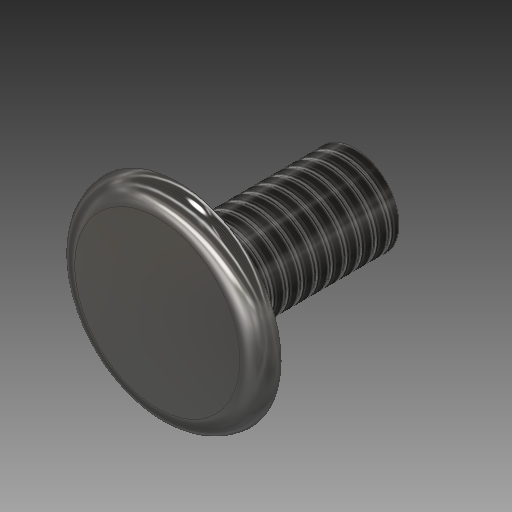
# Autodesk Inventor part: ネジ低頭m3.06
Saved by Autodesk Inventor 2019 (Build 230136000, 136)
## iProperties
Part Number: ネジ低頭m3.06
Material: 鋼、高強度、低合金
Document SubType Name: Modeling
Designer: 雪村
Mass: 0.527061 g
Surface Area: 1.42086 cm^2
Volume: 0.0671415 cm^3
Density: 7.85 g/cm^3
Appearance: 鋼 - つや出し
Author: 雪村
Autodesk Inventor part; units mm, degrees
ref_plane "YZ Plane" through (0, 0, 0) normal (1, 0, 0) x (0, 1, 0)
ref_plane "XZ Plane" through (0, 0, 0) normal (0, 1, 0) x (-1, 0, 0)
ref_plane "XY Plane" through (0, 0, 0) normal (0, 0, 1) x (1, 0, 0)
sketch "スケッチ1" plane through (0, 0, 0) normal (0, 0, 1) x (1, 0, 0)
  circle A0 centre (0, 0) radius 3.5
  dimension "d0" = 7
  constraints: 1 centre point, 1 coincident
  measures "d0" diameter of A0
extrude "押し出し1" add sketch "スケッチ1" along normal blind 0.7
sketch "スケッチ2" plane through (0, 0, 0) normal (0, 0, -1) x (-1, 0, 0)
  circle A0 centre (0, 0) radius 1.5
  dimension "d3" = 3
  constraints: 1 centre point, 1 coincident
  measures "d3" diameter of A0
extrude "押し出し2" add sketch "スケッチ2" along normal blind 6
thread "ねじ1" size "M3x0.5" class "6g" standard "ANSI Metric M Profile" full length
fillet "フィレット1" radius 0.7 1 edges at (-3.5, 0, 0.7)
